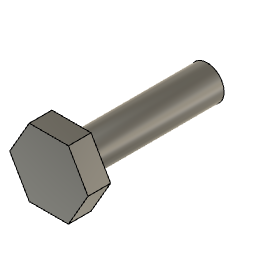
_Bolt & Nut.9ea0a2f4-d151-43dc-aaf8-f972b4006c54 (Autodesk Fusion 360 design; units mm, degrees)
Autodesk Fusion 360 part; units mm, degrees
sketch "Sketch1" plane through (0, 0, 0) normal (0, 1, 0) x (1, 0, 0)
  circle A0 centre (0, 0) radius 1.5
  line L0 (-1.7321, 3) -> (-3.4641, 0)
  line L1 (-3.4641, 0) -> (-1.7321, -3)
  line L2 (-1.7321, -3) -> (1.7321, -3)
  line L3 (1.7321, -3) -> (3.4641, 0)
  line L4 (3.4641, 0) -> (1.7321, 3)
  line L5 (1.7321, 3) -> (-1.7321, 3)
  dimension "d1" = 3
  dimension "d2" = 6
  constraint coincident A0.centre origin
  constraint horizontal L2
  measures "d1" diameter of A0
  measures "d2" distance of L2 L5
extrude "Extrude1" add sketch "Sketch1" along normal blind 12 contours A0
extrude "Extrude2" add sketch "Sketch1" against normal blind 2 contours A0 | L0 L1 L2 L3 L4 L5
